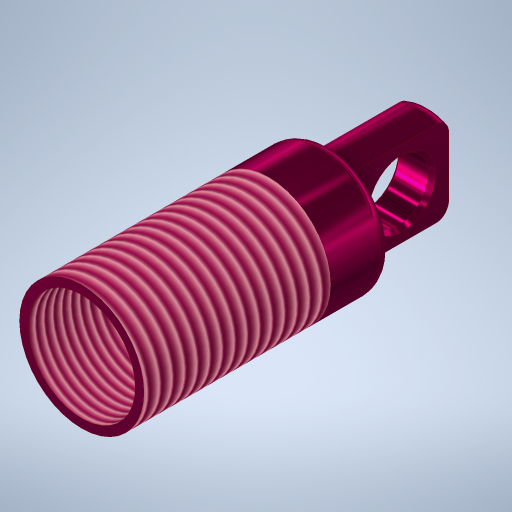
# Autodesk Inventor part: Shock Body 1.3 Length
Saved by Autodesk Inventor 2023.1 (Build 271208000, 208)
## iProperties
Created: 2019-11-29
Part Number: Shock Body 1.3 Length
Material: Generic
Document SubType Name: Modeling
Designer: Jopa
Density: 1 g/cm^3
Appearance: Anodized - Red
Author: Jopa
Autodesk Inventor part; units mm, degrees
ref_plane "YZ Plane" through (0, 0, 0) normal (1, 0, 0) x (0, 1, 0)
ref_plane "XZ Plane" through (0, 0, 0) normal (0, 1, 0) x (-1, 0, 0)
ref_plane "XY Plane" through (0, 0, 0) normal (0, 0, 1) x (1, 0, 0)
sketch "Sketch1" plane through (0, 0, 0) normal (0, 0, 1) x (1, 0, 0)
  circle A0 centre (0, 0) radius 6.35
  dimension "d0" = 12.7
  constraints: 1 centre point, 1 coincident
  measures "d0" diameter of A0
extrude "Extrusion1" add sketch "Sketch1" along normal blind 25.4
shell "Shell1" thickness 0.889 removed faces 1 at (-1.8127, -0.4771, 25.4)
fillet "Fillet1" radius 1.27 1 edges at (-6.35, 0, 0)
sketch "Sketch2" plane through (0, 0, 0) normal (0, 0, -1) x (-1, 0, 0)
  circle A0 centre (0, 0) radius 4.7625
  dimension "d5" = 9.525
  constraints: 1 centre point, 1 coincident
  measures "d5" diameter of A0
extrude "Extrusion2" add sketch "Sketch2" along normal blind 10.16
sketch "Sketch3" plane through (0, 0, -10.16) normal (0, 0, -1) x (-1, 0, 0)
  circle A0 centre (0, 0) radius 4.7625 projected
  circle A1 centre (0, 0) radius 4.7625 projected
  line L0 (-1.905, 4.3649) -> (-1.905, -4.3649)
  line L1 (1.905, 4.3649) -> (1.905, -4.3649)
  line L2 (0, -8.89) -> (0, 8.89) construction
  line L3 (8.89, 0) -> (-8.89, 0) construction
  circle A2 centre (0, 0) radius 4.7625 projected
  circle A3 centre (0, 0) radius 4.7625
  line L4 (-1.905, -4.3649) -> (-1.905, 4.3649)
  line L5 (1.905, 4.3649) -> (1.905, -4.3649)
  dimension "d8" = 3.81
  constraints: 8 end point, 5 point on circle, 3 equal length, 1 coincident, 1 vertical, 6 other
  measures "d8" distance between parallel lines of L1 L0
extrude "Extrusion3" cut sketch "Sketch3" against normal up to surface (10.16 mm away) contours A0 L1 | L0 A0
sketch "Sketch4" plane through (-1.905, -4.3649, -10.16) normal (-1, 0, 0) x (0, 0, 1)
  line L0 (-7.112, 4.3649) -> (42.672, 4.3649) projected
  line L1 (0, 0) -> (0, 8.7298) projected
  circle A0 centre (4.7625, 4.3649) radius 3.048
  point P0 (10.16, 4.3649)
  dimension "d11" = 6.096
  dimension "d12" = 4.7625
  constraints: 1 centre point, 1 point on line
  measures "d11" diameter of A0
  measures "d12" distance from line of L1 A0.centre
extrude "Extrusion4" cut sketch "Sketch4" along normal through all both and the other way through all
chamfer "Chamfer1" distance 0.381 angle 45 2 edges at (1.905, 0, -8.4455) (-1.905, 0, -8.4455)
fillet "Fillet2" radius 1.27 2 edges at (0, -4.7625, -10.16) (0, 4.7625, -10.16)
thread "Thread1" size "1/2-20 UNF" class "1A" standard "ANSI Unified Screw Threads" length 19.05
thread "Thread2" size "7/16-28 UNEF" class "2B" standard "ANSI Unified Screw Threads" length 9.525
body "Solid1"
